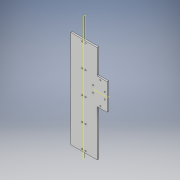
# Autodesk Inventor part: Backhoe to Frame Mount
Saved by Autodesk Inventor 2019 (Build 230136000, 136)
## iProperties
Created: 2018-11-29
Part Number: Backhoe to Frame Mount
Material: Generic
Document SubType Name: Modeling
Designer: Alex Barnett
Density: 1 g/cm^3
Appearance: Default
Author: Alex Barnett
Autodesk Inventor part; units mm, degrees
ref_plane "YZ Plane" through (0, 0, 0) normal (1, 0, 0) x (0, 1, 0)
ref_plane "XZ Plane" through (0, 0, 0) normal (0, 1, 0) x (-1, 0, 0)
ref_plane "XY Plane" through (0, 0, 0) normal (0, 0, 1) x (1, 0, 0)
sketch "Sketch1" plane through (0, 0, 0) normal (0, 0, 1) x (1, 0, 0)
  line L0 (0, 0) -> (101.6, 0)
  line L1 (101.6, 0) -> (101.6, 373.888)
  line L2 (101.6, 373.888) -> (0, 373.888)
  line L3 (0, 373.888) -> (0, 0)
  dimension "d0" = 101.6
  dimension "d1" = 373.888
  constraints: 8 end point, 2 parallel, 1 horizontal, 1 perpendicular
  measures "d0" distance of L2.end L1.end
  measures "d1" distance of L1.end L0.end
extrude "Extrusion1" add sketch "Sketch1" against normal blind 6.35
sketch "Sketch2" plane through (0, 0, 0) normal (0, 0, 1) x (1, 0, 0)
  line L0 (101.6, 0) -> (101.6, 373.888) projected
  line L1 (50.3784, 186.944) -> (-65.1556, 186.944) construction
  line L2 (0, 228.5746) -> (-60.1541, 228.5746) construction
  line L3 (101.6, 279.3746) -> (139.7, 279.3746)
  line L4 (139.7, 279.3746) -> (139.7, 177.7746)
  line L5 (139.7, 177.7746) -> (101.6, 177.7746)
  line L6 (101.6, 177.7746) -> (101.6, 279.3746)
  line L7 (0, 0) -> (101.6, 0) construction
  line L8 (101.6, 373.888) -> (0, 373.888) construction
  point P0 (101.6, 228.5746)
  dimension "d50" = 41.6306
  dimension "d51" = 38.1
  dimension "d52" = 101.6
  dimension "d53" = 373.888
  dimension "d54" = 186.944
  constraints: 12 end point, 3 horizontal, 2 parallel, 2 point on line, 1 midpoint, 1 perpendicular
  measures "d50" distance between parallel lines of L1 L2
  measures "d51" distance of L4.end L5.end
  measures "d52" distance of L3.end L4.end
  measures "d53" distance between parallel lines of L7 L8
  measures "d54" distance between parallel lines of L7 L1
extrude "Extrusion2" add sketch "Sketch2" against normal blind 6.35
fillet "Fillet1" radius 3.175 1 edges at (101.6, 279.3746, -3.175)
fillet "Fillet2" radius 3.175 1 edges at (101.6, 177.7746, -3.175)
sketch "Sketch3" plane through (0, 0, 0) normal (0, 0, 1) x (1, 0, 0)
  line L0 (101.6, 0) -> (101.6, 174.5996) projected
  line L1 (0, 0) -> (101.6, 0) projected
  point P0 (44.45, 7.62)
  point P1 (101.6, 132.969)
  point P2 (101.6, 180.594)
  dimension "d11" = 57.15
  dimension "d12" = 7.62
  measures "d11" distance from line of L0 point (44.45, 7.62)
  measures "d12" distance from line of L1 point (44.45, 7.62)
hole "Hole1" at (44.45, 7.62, 0) direction (0, 0, -1) diameter 5.08 end through all
ref_plane "Work Plane1" through (50.8, 0, 0) normal (-1, 0, 0) x (0, 0, 1)
pattern_linear "Rectangular Pattern1" count 2 spacing 12.7 along (1, 0, 0) count 5 spacing 89.662 along (0, 1, 0) of "Hole1"
ref_plane "Work Plane4" through (139.7, 228.5746, -6.35) normal (0, -1, 0) x (1, 0, 0)
sketch "Sketch6" plane through (0, 0, 0) normal (0, 0, 1) x (1, 0, 0)
  line L0 (139.7, 279.3746) -> (139.7, 177.7746) construction
  line L1 (139.7, 177.7746) -> (104.775, 177.7746) construction
  point P0 (0, 0)
  point P1 (114.3, 185.3946)
  dimension "d56" = 25.4
  dimension "d57" = 7.62
  measures "d56" distance from line of L0 point (114.3, 185.395)
  measures "d57" distance from line of L1 point (114.3, 185.395)
hole "Hole4" at (114.3, 185.3946, 0) direction (0, 0, -1) diameter 5.08 end through all
mirror "Mirror3" about plane through (139.7, 228.5746, -6.35) normal (0, -1, 0) of "Hole4"
sketch "Sketch7" plane through (0, 0, 0) normal (0, 0, 1) x (1, 0, 0)
  line L0 (0, 373.888) -> (0, 0) construction
  line L1 (167.64, 228.5746) -> (-27.94, 228.5746) projected
  point P0 (86.2584, 241.2746)
  dimension "d65" = 86.2584
  dimension "d73" = 12.7
  measures "d65" distance from line of L0 point (86.258, 241.275)
  measures "d73" distance from line of point (86.258, 241.275) L1
hole "Hole5" at (86.2584, 241.2746, 0) direction (0, 0, -1) diameter 5.08 end through all
pattern_linear "Rectangular Pattern3" count 2 spacing 25.4 along (0, -1, 0) count 2 spacing 44.45 along (1, 0, 0) of "Hole5"
body "Solid1"
